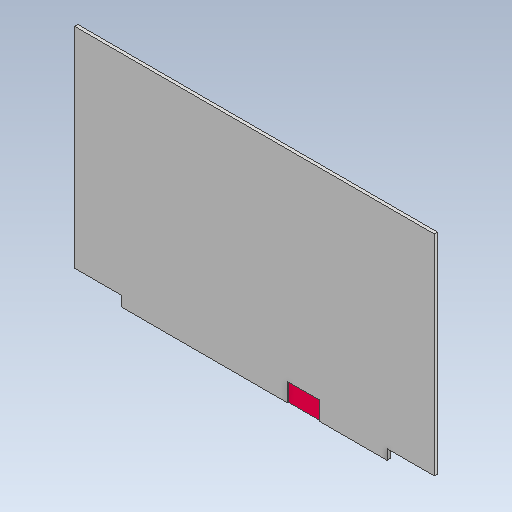
# Autodesk Inventor part: NV173FHM-N4G V8.0
Saved by Autodesk Inventor 2021.2 (Build 252289000, 289)
## iProperties
Created: 2022-11-28
Part Number: NV173FHM-N4G V8.0
Material: Типовые
Document SubType Name: Modeling
Designer: Voodoo
Mass: 311.815 g
Surface Area: 1881.58 cm^2
Volume: 311.815 cm^3
Density: 1 g/cm^3
Appearance: По умолчанию
Author: Voodoo
Autodesk Inventor part; units mm, degrees
ref_plane "YZ Plane" through (0, 0, 0) normal (1, 0, 0) x (0, 1, 0)
ref_plane "XZ Plane" through (0, 0, 0) normal (0, 1, 0) x (-1, 0, 0)
ref_plane "XY Plane" through (0, 0, 0) normal (0, 0, 1) x (1, 0, 0)
sketch "Эскиз1" plane through (0, 0, 0) normal (0, 0, 1) x (1, 0, 0)
  line L0 (0, 0) -> (390, 0)
  line L1 (390, 0) -> (390, 227)
  line L2 (390, 227) -> (0, 227)
  line L3 (0, 227) -> (0, 0)
  line L4 (4, 223) -> (386, 223)
  line L5 (386, 223) -> (386, 8)
  line L6 (386, 8) -> (4, 8)
  line L7 (4, 8) -> (4, 223)
  line L8 (51.2, 0) -> (338.8, 0)
  line L9 (338.8, 0) -> (338.8, -11)
  line L10 (338.8, -11) -> (51.2, -11)
  line L11 (51.2, -11) -> (51.2, 0)
  line L12 (195, 8) -> (195, 37.2602)
  point P0 (195, 223)
  point P1 (195, 227)
  point P2 (195, -11)
  dimension "d0" = 390
  dimension "d1" = 227
  dimension "d2" = 382
  dimension "d3" = 215
  dimension "d4" = 4
  dimension "d5" = 8
  dimension "d6" = 4
  dimension "d7" = 238
  dimension "d9" = 287.6
  constraints: 26 end point, 6 parallel, 4 midpoint, 3 horizontal, 3 perpendicular, 2 vertical alignment, 1 point on line, 1 vertical
  measures "d0" distance of L1.end L2.end
  measures "d1" distance of L2.end L0.start
  measures "d2" distance of L4.start L4.end
  measures "d3" distance of L6.end L4.start
  measures "d4" distance between parallel lines of L2 L4
  measures "d5" distance between parallel lines of L6 L0
  measures "d6" distance between parallel lines of L7 L3
  measures "d7" distance between parallel lines of L2 L10
  measures "d9" distance of L9.end L10.end
extrude "Выдавливание1" add sketch "Эскиз1" along normal blind 3.5
sketch "Эскиз2" plane through (0, 0, 3.5) normal (0, 0, 1) x (1, 0, 0)
  line L0 (0, 0) -> (51.2, 0) projected
  line L1 (51.2, 0) -> (51.2, -11) projected
  line L2 (51.2, -11) -> (338.8, -11) projected
  line L3 (338.8, -11) -> (338.8, 0) projected
  line L4 (338.8, 0) -> (390, 0) projected
  line L5 (390, 0) -> (390, 227) projected
  line L6 (390, 227) -> (0, 227) projected
  line L7 (0, 227) -> (0, 0) projected
  line L8 (386, 223) -> (386, 8) projected
  line L9 (386, 8) -> (4, 8) projected
  line L10 (4, 8) -> (4, 223) projected
  line L11 (4, 223) -> (386, 223) projected
extrude "Выдавливание2" add sketch "Эскиз2" against normal blind 3.4 contours L8 L9 L10 L11
sketch "Эскиз3" plane through (0, 0, 0) normal (0, 0, -1) x (-1, 0, 0)
  line L0 (0, 0) -> (-51.2, 0) projected
  line L1 (0, 227) -> (0, 0) projected
  line L2 (-390, 227) -> (0, 227) projected
  line L3 (-390, 0) -> (-390, 227) projected
  line L4 (-338.8, 0) -> (-390, 0) projected
  line L5 (-338.8, -11) -> (-338.8, 0) projected
  line L6 (-51.2, -11) -> (-338.8, -11) projected
  line L7 (-51.2, 0) -> (-51.2, -11) projected
  line L8 (-386, 223) -> (-386, 8) projected
  line L9 (-4, 223) -> (-386, 223) projected
  line L10 (-4, 8) -> (-4, 223) projected
  line L11 (-386, 8) -> (-4, 8) projected
  line L12 (-195, -11) -> (-195, 1.1845)
  line L13 (-255.24, 5) -> (-230.3, 5)
  line L14 (-230.3, 5) -> (-230.3, 3)
  line L15 (-230.3, 3) -> (-255.24, 3)
  line L16 (-255.24, 3) -> (-255.24, 5)
  line L17 (-338.98, 5) -> (-314.04, 5)
  line L18 (-314.04, 5) -> (-314.04, 3)
  line L19 (-314.04, 3) -> (-338.98, 3)
  line L20 (-338.98, 3) -> (-338.98, 5)
  line L21 (-134.76, 5) -> (-159.7, 5)
  line L22 (-159.7, 5) -> (-159.7, 3)
  line L23 (-159.7, 3) -> (-134.76, 3)
  line L24 (-134.76, 3) -> (-134.76, 5)
  line L25 (-51.02, 5) -> (-75.96, 5)
  line L26 (-75.96, 5) -> (-75.96, 3)
  line L27 (-75.96, 3) -> (-51.02, 3)
  line L28 (-51.02, 3) -> (-51.02, 5)
  point P0 (-314.04, 4)
  point P1 (-255.24, 4)
  point P2 (-75.96, 4)
  point P3 (-134.76, 4)
  dimension "d14" = 24.94
  dimension "d15" = 35.3
  dimension "d16" = 3
  dimension "d17" = 2
  dimension "d18" = 2
  dimension "d19" = 24.94
  dimension "d20" = 58.8
  constraints: 34 end point, 10 symmetric about line, 4 parallel, 4 point on line, 3 midpoint, 2 horizontal, 2 perpendicular, 1 horizontal alignment, 1 vertical
  measures "d14" distance of L14.end L15.end
  measures "d15" distance from line of L14.end L12
  measures "d16" distance between parallel lines of L11 L13
  measures "d17" distance of L13.end L14.end
  measures "d18" distance between parallel lines of L17 L19
  measures "d19" distance of L18.end L19.end
  measures "d20" distance of point (-255.24, 4) point (-314.04, 4)
extrude "Выдавливание3" cut sketch "Эскиз3" against normal blind 1 contours L13 L14 L15 L16 | L17 L18 L19 L20 | L24 L23 L22 L21 | L28 L27 L26 L25
sketch "Эскиз5" plane through (0, 0, 3.5) normal (0, 0, 1) x (1, 0, 0)
  line L0 (0, 0) -> (51.2, 0) projected
  line L1 (51.2, 0) -> (51.2, -11) projected
  line L2 (51.2, -11) -> (338.8, -11) projected
  line L3 (338.8, -11) -> (338.8, 0) projected
  line L4 (338.8, 0) -> (390, 0) projected
  line L5 (390, 0) -> (390, 227) projected
  line L6 (390, 227) -> (0, 227) projected
  line L7 (0, 227) -> (0, 0) projected
  line L8 (230.5, -11) -> (265.5, -11)
  line L9 (265.5, -11) -> (265.5, 9)
  line L10 (265.5, 9) -> (230.5, 9)
  line L11 (230.5, 9) -> (230.5, -11)
  dimension "d23" = 124.5
  dimension "d24" = 20
  dimension "d25" = 35
  constraints: 8 end point, 2 parallel, 1 collinear, 1 horizontal, 1 perpendicular
  measures "d23" distance between parallel lines of L5 L9
  measures "d24" distance of L8.end L9.end
  measures "d25" distance of L9.end L10.end
extrude "Выдавливание4" cut sketch "Эскиз5" against normal blind 1 contours L11 L10 L9 L2
equation "\"d19\" = d14"
